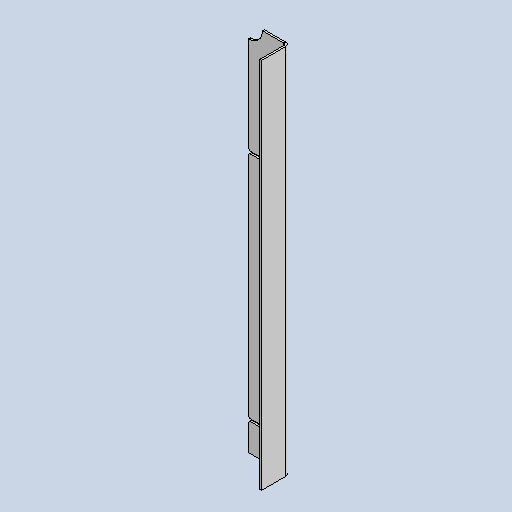
# Autodesk Inventor part: GBK 0104 stringer 3_Dummy
Saved by Autodesk Inventor 2026.2 (Build 302298010, 298A)
## iProperties
Created: 2026-05-07
Part Number: GBK 0104 stringer 3_Dummy
Material: Steel
Document SubType Name: Sheet Metal
Designer: admin
Mass: 3406.9 g
Surface Area: 2251.08 cm^2
Volume: 434 cm^3
Density: 7.85 g/cm^3
Flat Pattern Width: 13.7048 cm
Flat Pattern Length: 79.8 cm
Flat Pattern Area: 1093.64 cm^2
Sheet Metal Rule: Default_mm
Sheet Metal Width: 137,048 mm
Sheet Metal Length: 798,000 mm
Sheet Metal Area: 109364,134 mm^2
Appearance: Default
Author: admin
Autodesk Inventor part; units mm, degrees
ref_plane "YZ Plane" through (0, 0, 0) normal (1, 0, 0) x (0, 1, 0)
ref_plane "XZ Plane" through (0, 0, 0) normal (0, 1, 0) x (-1, 0, 0)
ref_plane "XY Plane" through (0, 0, 0) normal (0, 0, 1) x (1, 0, 0)
sketch "Sketch1" plane through (0, 0, 0) normal (0, 0, 1) x (1, 0, 0)
  line L0 (0, 0) -> (-84, 0)
  line L1 (-84, 0) -> (-84, -1490)
  line L2 (-84, -1490) -> (0, -1490)
  line L3 (0, -1490) -> (0, 0)
  line L4 (-84, -1390) -> (-40, -1390)
  line L5 (-40, -1390) -> (-40, -1385)
  line L6 (-40, -1385) -> (-84, -1385)
  line L7 (-84, -1385) -> (-84, -1390)
  line L8 (-84, -893.3333) -> (-40, -893.3333)
  line L9 (-40, -893.3333) -> (-40, -888.3333)
  line L10 (-40, -888.3333) -> (-84, -888.3333)
  line L11 (-84, -888.3333) -> (-84, -893.3333)
  line L12 (-84, -396.6667) -> (-40, -396.6667)
  line L13 (-40, -396.6667) -> (-40, -391.6667)
  line L14 (-40, -391.6667) -> (-84, -391.6667)
  line L15 (-84, -391.6667) -> (-84, -396.6667)
  circle A0 centre (-84, -155) radius 30
  line L16 (-84, -953) -> (0, -953)
  line L17 (-84, -155) -> (0, -155)
  point P0 (-84, -391.6667)
  point P1 (-84, -396.6667)
  point P2 (-84, -888.3333)
  point P3 (-84, -893.3333)
  point P4 (-84, -1385)
  point P5 (-84, -125)
  point P6 (-84, -185)
  point P7 (-54, -155)
  dimension "d0" = 1490
  dimension "d1" = 84
  dimension "d2" = 5
  dimension "d4" = 100
  dimension "d7" = 496.6667
  dimension "d23" = 40
  dimension "d28" = 60
  dimension "d29" = 1335
  dimension "d30" = 953
  measures "d0" distance of L1.end L0.end
  measures "d1" distance of L1.end L2.end
  measures "d2" distance of L4.end L5.end
  measures "d4" distance between parallel lines of L2 L4
  measures "d7" distance of L4.start L8.start
  measures "d23" distance between parallel lines of L3 L5
  measures "d28" diameter of A0
  measures "d29" distance from line of L17.start L2
  measures "d30" distance between parallel lines of L16 L0
extrude "Plate1" add sketch "Sketch1" along normal blind 4 contours L3 L16 L1 L8 L9 L10 L12 L13 L14 A0 L17
sketch "Sketch2" plane through (-4, -155, 0) normal (1, 0, 0) x (0, 1, 0)
  line L0 (-798, 0) -> (0, 0)
  line L1 (0, 0) -> (0, 60)
  line L2 (0, 60) -> (-798, 60)
  line L3 (-798, 60) -> (-798, 0)
  constraints: 6 end point, 1 horizontal, 1 perpendicular, 1 vertical
edge flange "Flange1" height 60 angle 90 thickness 4 bend radius 4 thickness toward (1, 0, 0) relief tear relief width 4 relief depth 2 edges at (0, -554, 4) wall of the first edge with corners at (-4, -953, 0) (-4, -155, 0) (-4, -155, 60) (-4, -953, 60)
bend "Bend1"
corner "Corner1"
chamfer "Corner Chamfer1" distance 3 angle 45 4 edges at (-84, -893.3333, 2) (-84, -888.3333, 2) (-84, -391.6667, 2) (-84, -396.6667, 2)
equation "\"d0\" = Стрингер_длина"
equation "\"d2\" = паз_под_стрингер_толщина"
equation "\"d7\" = Шаг_шпангоутов"
equation "\"d28\" = 2 * радиус_выреза_под_сварку"
equation "\"d12\" = Thickness"
equation "\"d13\" = BendReliefWidth"
equation "\"d14\" = BendReliefDepth"
equation "\"d15\" = MinimumRemnant"
equation "\"d16\" = TransitionRadius"
equation "\"d17\" = ребро_усилителей"
equation "\"d19\" = BendRadius"
equation "\"d20\" = CornerReliefSize"
equation "\"d21\" = GapSize"
equation "\"d22\" = JacobiRadiusSize"
equation "\"BendRadius\" = Thickness"
equation "\"BendReliefWidth\" = Thickness"
equation "\"BendReliefDepth\" = 0.5 * Thickness"
equation "\"CornerReliefSize\" = 4 * Thickness"
equation "\"MinimumRemnant\" = 2 * Thickness"
equation "\"TransitionRadius\" = BendRadius"
equation "\"JacobiRadiusSize\" = BendRadius"
equation "\"GapSize\" = Thickness"
equation "\"Стрингер_длина\" = 1490"
equation "\"паз_под_стрингер_толщина\" = 5"
equation "\"Шаг_шпангоутов\" = 496.666667"
equation "\"радиус_выреза_под_сварку\" = 30"
equation "\"Thickness\" = 4"
equation "\"ребро_усилителей\" = 60"
body "Solid1"
